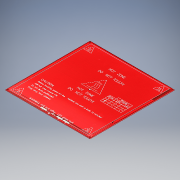
# Autodesk Inventor part: HotBed_PCB_LM6020
Saved by Autodesk Inventor 2020.3 (Build 243373000, 373)
## iProperties
Created: 2020-05-12
Part Number: HotBed_PCB_LM6020
Material: Copper
Document SubType Name: Modeling
Designer: rah75
Density: 8.94 g/cm^3
Appearance: Satin -Light Red
Author: rah75
Autodesk Inventor part; units mm, degrees
ref_plane "YZ Plane" through (0, 0, 0) normal (1, 0, 0) x (0, 1, 0)
ref_plane "XZ Plane" through (0, 0, 0) normal (0, 1, 0) x (-1, 0, 0)
ref_plane "XY Plane" through (0, 0, 0) normal (0, 0, 1) x (1, 0, 0)
sketch "Sketch1" plane through (0, 0, 0) normal (0, 1, 0) x (-1, 0, 0)
  line L0 (107, -107) -> (-107, -107)
  line L1 (-107, -107) -> (-107, 107)
  line L2 (-107, 107) -> (107, 107)
  line L3 (107, 107) -> (107, -107)
  line L4 (107, -107) -> (-107, 107) construction
  line L5 (-107, -107) -> (107, 107) construction
  line L6 (104.5, 104.5) -> (-104.5, 104.5) construction
  line L7 (-104.5, 104.5) -> (-104.5, -104.5) construction
  line L8 (-104.5, -104.5) -> (104.5, -104.5) construction
  line L9 (104.5, -104.5) -> (104.5, 104.5) construction
  line L10 (104.5, 104.5) -> (-104.5, -104.5) construction
  line L11 (-104.5, 104.5) -> (104.5, -104.5) construction
  circle A0 centre (104.5, -104.5) radius 1.6
  circle A1 centre (-104.5, -104.5) radius 1.6
  circle A2 centre (-104.5, 104.5) radius 1.6
  circle A3 centre (104.5, 104.5) radius 1.6
  point P0 (0, 0)
  dimension "d0" = 214
  dimension "d1" = 214
  dimension "d2" = 209
  dimension "d3" = 209
  dimension "d4" = 3.2
  dimension "d5" = 3.2
  dimension "d6" = 3.2
  dimension "d7" = 3.2
  constraints: 24 end point, 4 centre point, 4 coincident, 4 midpoint, 4 parallel, 2 horizontal, 2 perpendicular
  measures "d0" distance of L1.end L2.end
  measures "d1" distance of L0.end L1.end
  measures "d2" distance of L8.end L7.end
  measures "d3" distance of L7.end L6.end
  measures "d4" diameter of A0
  measures "d5" diameter of A1
  measures "d6" diameter of A2
  measures "d7" diameter of A3
extrude "Extrusion1" add sketch "Sketch1" along normal mid plane 2
sketch "Sketch2" plane through (0, 1, 0) normal (0, 1, 0) x (1, 0, 0)
  line L0 (58.5536, -54.476) -> (-58.5536, -54.476)
  line L1 (-58.5536, -54.476) -> (-58.5536, 54.476)
  line L2 (-58.5536, 54.476) -> (58.5536, 54.476)
  line L3 (58.5536, 54.476) -> (58.5536, -54.476)
  line L4 (58.5536, -54.476) -> (-58.5536, 54.476) construction
  line L5 (-58.5536, -54.476) -> (58.5536, 54.476) construction
  line L6 (107, 107) -> (-107, 107) projected
  line L7 (-107, 107) -> (106.5967, 107.4017) construction
  line L8 (106.5967, 107.4017) -> (107, -107) construction
  line L9 (107, -107) -> (-106.5967, -107.4017) construction
  line L10 (-106.5967, -107.4017) -> (-107, 107) construction
  point P0 (0, 0)
  constraints: 12 end point, 2 midpoint, 2 parallel, 1 coincident, 1 horizontal, 1 perpendicular, 2 other
decal "Decal1"
body "Solid1"
